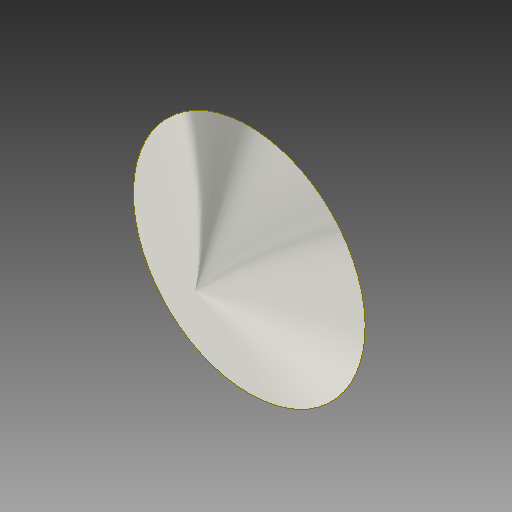
# Autodesk Inventor part: mirror2
Saved by Autodesk Inventor 2020 (Build 240168000, 168)
## iProperties
Created: 2024-12-06
Part Number: mirror2
Material: Типовые
Document SubType Name: Modeling
Designer: Ivan
Density: 1 g/cm^3
Appearance: Серебро
Author: Ivan
Autodesk Inventor part; units mm, degrees
ref_plane "YZ Plane" through (0, 0, 0) normal (1, 0, 0) x (0, 1, 0)
ref_plane "XZ Plane" through (0, 0, 0) normal (0, 1, 0) x (-1, 0, 0)
ref_plane "XY Plane" through (0, 0, 0) normal (0, 0, 1) x (1, 0, 0)
sketch "Эскиз1" plane through (0, 0, 0) normal (1, 0, 0) x (0, 1, 0)
  line L0 (-97.1998, 152.9865) -> (97.1998, 152.9865) projected
  line L1 (27.0115, 58.2424) -> (-26.9885, 58.2424) projected
  line L2 (-4.8441, 44.0424) -> (4.8559, 44.0424) construction
  line L3 (0.0115, 216.6365) -> (-2699.9885, 216.6365)
  ellipse E0 centre (-65.8475, 190.1365) end of major axis (-65.8475, 216.6365) minor radius 18.7383 projected
  line L4 (0.0115, 58.2424) -> (0.0115, 216.6365) construction
  line L5 (27.0115, 58.2424) -> (-26.9885, 58.2424) construction
  line L6 (-2699.9885, 216.6365) -> (-2699.9885, 96.6365)
  line L7 (0.0115, 58.2424) -> (0.0115, -1.5) construction
  line L8 (-6.7941, 43.9424) -> (6.8059, 43.9424) projected
  line L9 (27.0115, 15.7485) -> (-26.9885, 15.7485)
  line L10 (-26.9885, 15.7485) -> (0.0115, 28.3712)
  line L11 (27.0115, 15.7485) -> (0.0115, 28.3712)
  line L12 (-4.6441, 44.0424) -> (-26.8073, 15.8332) construction
  line L13 (4.6559, 44.0424) -> (-3.4855, 54.4048) construction
  line L14 (-26.8073, 15.8332) -> (-24.4759, 10.8463) construction
  line L15 (-62.6653, 16.9171) -> (-26.8073, 15.8332) construction
  line L16 (-62.6653, 16.9171) -> (-2699.9885, 96.6365)
  line L17 (-0.0885, 44.0424) -> (-0.0885, 28.3245) construction
  line L18 (0.0115, 28.3712) -> (0.0115, 15.7485)
  line L19 (-0.0885, 28.3245) -> (-0.563, 29.3395) construction
  line L20 (-12.149, 38.4041) -> (-0.0885, 28.3245) construction
  line L21 (-12.149, 38.4041) -> (-119.3337, 127.9837)
  circle A0 centre (-144, 170) radius 37
  point P0 (0.0115, 47.4305)
  dimension "d10" = 2700
  dimension "d11" = 120
  dimension "d12" = 218.1365
  dimension "d13" = 45.4424
  dimension "d16" = 0.2
  dimension "d17" = 0.1
  dimension "d19" = 0.2
  dimension "d20" = 76.312
  dimension "d21" = 38.156
  dimension "d25" = 0
  dimension "d26" = 54
  dimension "d32" = 74
  dimension "d34" = 0.2
  dimension "d35" = 19.0592
  constraints: 34 end point, 6 point on line, 4 midpoint, 3 perpendicular, 2 collinear, 2 horizontal, 2 symmetric about line, 2 vertical, 1 centre point, 1 equal length, 1 other
  measures "d10" distance of L3.start L3.end
  measures "d11" distance of L3.end L6.end
  measures "d12" distance of L7.end L3.start
  measures "d13" distance from line of L7.end L8
  measures "d16" distance of L12.start L2.start
  measures "d17" distance from line of L7 L17.start
  measures "d19" distance of L13.start L2.end
  measures "d20" angle of L12 L13
  measures "d21" angle of L12 L7
  measures "d25" angle of L17 L7
  measures "d26" distance of L9.start L9.end
  measures "d32" diameter of A0
  measures "d34" distance from line of L14 L9.end
  measures "d35" distance of L10.end point (0.012, 47.43)
revolve "Вращение1" add sketch "Эскиз1" angle 360 about axis through (0, 0.0115, 58.2424) along (0, 0, -1) contours L9 L10 L18
sketch "Эскиз3" plane through (0, 0, 0) normal (1, 0, 0) x (0, 1, 0)
  point P0 (0, 0)
equation "\"d19\" = d16"
equation "\"d21\" = 0.5 * d20"
